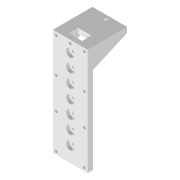
# Autodesk Inventor part: 30_Linear_Captive_Nema8_Base
Saved by Autodesk Inventor 2022 (Build 260153000, 153)
## iProperties
Created: 2022-12-17
Part Number: 30_Linear_Captive_Nema8_Base
Material: Generisch
Document SubType Name: Modeling
Designer: diederichbenedict
Density: 1 g/cm^3
Appearance: Vorgabe
Author: diederichbenedict
Autodesk Inventor part; units mm, degrees
ref_plane "YZ Plane" through (0, 0, 0) normal (1, 0, 0) x (0, 1, 0)
ref_plane "XZ Plane" through (0, 0, 0) normal (0, 1, 0) x (-1, 0, 0)
ref_plane "XY Plane" through (0, 0, 0) normal (0, 0, 1) x (1, 0, 0)
ref_plane "Arbeitsebene1" through (0, 0, 0) normal (0, 0, 1) x (1, 0, 0)
sketch "Skizze1" plane through (0, 0, 0) normal (0, 0, 1) x (1, 0, 0)
  circle A0 centre (0.1, 41.9017) radius 1.75 projected
  circle A1 centre (0.1, 29.4017) radius 1.75 projected
  circle A2 centre (0.1, 16.9017) radius 1.75 projected
  circle A3 centre (0.1, 4.4017) radius 1.75 projected
  line L0 (6.05, 0) -> (-6.05, 0) projected
  line L1 (6.05, 0) -> (6.05, 50) projected
  line L2 (6.05, 50) -> (-6.05, 50) projected
  line L3 (-6.05, 0) -> (-6.05, 50) projected
  line L4 (13.5, 40.6086) -> (13.5, 8.2086) projected
  line L5 (-13.5, 40.6086) -> (-13.5, 8.2086) projected
  line L6 (13.5, -9.8404) -> (-13.3608, -9.8404)
  line L7 (-13.3608, -9.8404) -> (-13.3608, 90.1596)
  line L8 (-13.3608, 90.1596) -> (13.5, 90.1596)
  line L9 (13.5, 90.1596) -> (13.5, -9.8404)
  line L10 (-13.3608, 90.1596) -> (-16.2, 90.1596)
  line L11 (-16.2, 90.1596) -> (-16.2, -9.8404)
  line L12 (-16.2, -9.8404) -> (-13.3608, -9.8404)
  line L13 (-13.3608, -9.8404) -> (-13.3608, 90.1596)
  line L14 (13.5, -9.8404) -> (16.2, -9.8404)
  line L15 (16.2, -9.8404) -> (16.2, 90.1596)
  line L16 (16.2, 90.1596) -> (13.5, 90.1596)
  line L17 (13.5, 90.1596) -> (13.5, -9.8404)
  point P0 (0, 0)
  dimension "d0" = 100
  dimension "d34" = 27
  dimension "d35" = 2.7
  dimension "d36" = 2.7
  constraints: 24 end point, 6 parallel, 3 horizontal, 3 perpendicular, 1 point on line
  measures "d0" distance of L6.end L7.end
  measures "d34" distance from line of L9 L5.start
  measures "d35" distance between parallel lines of L5 L11
  measures "d36" distance between parallel lines of L15 L9
extrude "Extrusion1" add sketch "Skizze1" along normal blind 5 contours A0 | A1 | A2 | A3 | L0 L3 L2 L1 | L9 L16 L15 L14 L4 | L4 L9 L6 L7 L8 | L7 L12 L11 L10
sketch "Skizze2" plane through (0, 0, 0) normal (0, 0, -1) x (-1, 0, 0)
  line L0 (-13.5, 90.1596) -> (16.2, 90.1596)
  line L1 (16.2, 90.1596) -> (-16.2, 90.1596)
  line L2 (-16.2, 90.1596) -> (-16.1921, 85.1596)
  line L3 (-16.1921, 85.1596) -> (16.2, 85.1596)
  line L4 (16.2, 85.1596) -> (16.2, 90.1596)
  line L5 (13.3608, -9.8404) -> (-13.5, -9.8404)
  line L6 (-13.5, -9.8404) -> (-13.5, -4.8404)
  line L7 (-13.5, -4.8404) -> (13.3608, -4.8404)
  line L8 (13.3608, -4.8404) -> (13.3608, -9.8404)
  line L9 (-16.2, 90.1596) -> (16.2, 90.1596) projected
  point P0 (0, 0)
  dimension "d3" = 5
  dimension "d4" = 5
  constraints: 18 end point, 2 coincident, 1 parallel
  measures "d3" distance of L2.end L1.end
  measures "d4" distance of L5.end L6.end
extrude "Extrusion2" add sketch "Skizze2" along normal blind 32 contours L0 L4 L3 L2 L1
sketch "Skizze3" plane through (16.2, -9.8404, 5) normal (1, 0, 0) x (0, 0, -1)
  line L0 (5, 0) -> (5, 95) projected
  line L1 (5, 95) -> (37, 95) projected
  line L2 (37, 100) -> (37, 95) projected
  line L3 (37, 100) -> (0, 100) projected
  line L4 (0, 0) -> (0, 100) projected
  line L5 (37, 100) -> (37, 95) projected
  line L6 (37, 95) -> (5, 80.9723)
  line L7 (5, 95) -> (5, 5) projected
  line L8 (5, 0) -> (0, 0) projected
  point P0 (5, 9.8404)
  constraints: 2 end point, 1 point on line
extrude "Extrusion3" add sketch "Skizze3" against normal blind 5 contours L0 L1 L6
sketch "Skizze4" plane through (-16.2, -9.8404, 5) normal (-1, 0, 0) x (0, 0, 1)
  line L0 (-5, 95) -> (-5, 80.9723) projected
  line L1 (-37, 95) -> (-5, 95) projected
  line L2 (-37, 95) -> (-5, 80.9723) projected
  point P0 (-5, 9.8404)
extrude "Extrusion4" add sketch "Skizze4" against normal blind 5
sketch "Skizze5" plane through (11.2, 85.1596, -32) normal (0, -1, 0) x (1, 0, 0)
  circle A0 centre (-11.2, 4.1) radius 1.75 projected
  point P0 (-11.2, 32)
hole "Bohrung1" at (0, 85.1596, -27.9) direction (0, 1, 0) diameter 3.2 end through all counterbore diameter 6 counterbore depth 3
sketch "Skizze6" plane through (0, 0, 5) normal (0, 0, 1) x (1, 0, 0)
  circle A0 centre (0.1, 16.9017) radius 1.75 projected
  point P0 (0, 0)
hole "Bohrung2" at (0.1, 16.9017, 5) direction (0, 0, -1) diameter 3.2 end through all counterbore diameter 8 counterbore depth 3
pattern_linear "Rechteckige Anordnung1" count 6 spacing 12.5 along (0, 1, 0) count 2 spacing 12.5 along (0, -1, 0) of "Bohrung2"
sketch "Skizze7" plane through (-13.3608, 90.1596, 5) normal (0, 1, 0) x (1, 0, 0)
  arc A0 (19.4108, 9.1706) -> (19.209, 9.3127) centre (19.1621, 9.0317) ccw projected
  arc A1 (18.9122, 9.7059) -> (19.209, 9.3127) centre (19.9951, 10.2147) ccw projected
  arc A2 (18.9122, 9.7059) -> (18.7859, 9.8171) centre (18.694, 9.5854) ccw projected
  line L0 (18.7859, 9.8171) -> (18.2888, 9.8559) projected
  arc A3 (18.0608, 10.0745) -> (18.2888, 9.8559) centre (18.3083, 10.1044) ccw projected
  line L1 (18.0608, 10.0745) -> (18.0608, 10.5256) projected
  arc A4 (18.2884, 10.7739) -> (18.0608, 10.5256) centre (18.3101, 10.5256) ccw projected
  line L2 (18.2884, 10.7739) -> (18.6539, 10.8058) projected
  arc A5 (18.6539, 10.8058) -> (18.9122, 10.9588) centre (18.6817, 11.0536) ccw projected
  arc A6 (19.2562, 11.4767) -> (18.9122, 10.9588) centre (20.0633, 10.5674) ccw projected
  arc A7 (19.2562, 11.4767) -> (19.4108, 11.7) centre (19.1617, 11.7073) ccw projected
  line L3 (19.4108, 11.7) -> (19.4108, 12.3) projected
  line L4 (19.4108, 12.3) -> (18.9108, 12.8) projected
  line L5 (18.9108, 12.8) -> (7.8108, 12.8) projected
  line L6 (7.3108, 12.3) -> (7.8108, 12.8) projected
  line L7 (7.3108, 11.7) -> (7.3108, 12.3) projected
  arc A8 (7.3108, 11.7) -> (7.4655, 11.4767) centre (7.56, 11.7073) ccw projected
  arc A9 (7.8095, 10.9588) -> (7.4655, 11.4767) centre (6.6584, 10.5674) ccw projected
  arc A10 (7.8095, 10.9588) -> (8.0678, 10.8058) centre (8.04, 11.0536) ccw projected
  line L8 (8.4333, 10.7739) -> (8.0678, 10.8058) projected
  arc A11 (8.6608, 10.5256) -> (8.4333, 10.7739) centre (8.4116, 10.5256) ccw projected
  line L9 (8.6608, 10.0745) -> (8.6608, 10.5256) projected
  arc A12 (8.4328, 9.8559) -> (8.6608, 10.0745) centre (8.4134, 10.1044) ccw projected
  line L10 (7.9358, 9.8171) -> (8.4328, 9.8559) projected
  arc A13 (7.9358, 9.8171) -> (7.8095, 9.7059) centre (8.0277, 9.5854) ccw projected
  arc A14 (7.5127, 9.3127) -> (7.8095, 9.7059) centre (6.7266, 10.2147) ccw projected
  arc A15 (7.5127, 9.3127) -> (7.3108, 9.1706) centre (7.5596, 9.0317) ccw projected
  line L11 (7.3108, 5) -> (7.3108, 9.1706) projected
  line L12 (19.4108, 5) -> (7.3108, 5) projected
  line L13 (19.4108, 5) -> (19.4108, 9.1706) projected
  arc A16 (19.9108, 9.2672) -> (19.475, 9.7515) centre (19.1621, 9.0317) ccw
  arc A17 (19.3606, 9.9276) -> (19.475, 9.7515) centre (19.9951, 10.2147) ccw
  arc A18 (19.3606, 9.9276) -> (18.8795, 10.3114) centre (18.694, 9.5854) ccw
  line L14 (18.8795, 10.3114) -> (18.8155, 10.3163)
  arc A19 (18.8155, 10.3163) -> (19.3826, 10.7888) centre (18.6817, 11.0536) ccw
  arc A20 (19.5506, 11.0669) -> (19.3826, 10.7888) centre (20.0633, 10.5674) ccw
  arc A21 (19.5506, 11.0669) -> (19.9108, 11.6946) centre (19.1617, 11.7073) ccw
  line L15 (19.9108, 11.6946) -> (19.9108, 12.5071)
  line L16 (19.9108, 12.5071) -> (19.118, 13.3)
  line L17 (19.118, 13.3) -> (7.6037, 13.3)
  line L18 (7.6037, 13.3) -> (6.8108, 12.5071)
  line L19 (6.8108, 12.5071) -> (6.8108, 11.6946)
  arc A22 (6.8108, 11.6946) -> (7.1711, 11.0669) centre (7.56, 11.7073) ccw
  arc A23 (7.3391, 10.7888) -> (7.1711, 11.0669) centre (6.6584, 10.5674) ccw
  arc A24 (7.3391, 10.7888) -> (7.9062, 10.3163) centre (8.04, 11.0536) ccw
  line L20 (7.9062, 10.3163) -> (7.8422, 10.3114)
  arc A25 (7.8422, 10.3114) -> (7.3611, 9.9276) centre (8.0277, 9.5854) ccw
  arc A26 (7.2467, 9.7515) -> (7.3611, 9.9276) centre (6.7266, 10.2147) ccw
  arc A27 (7.2467, 9.7515) -> (6.8108, 9.2672) centre (7.5596, 9.0317) ccw
  line L21 (6.8108, 9.2672) -> (6.8108, 4.5)
  line L22 (6.8108, 4.5) -> (19.9108, 4.5)
  line L23 (19.9108, 4.5) -> (19.9108, 9.2672)
  point P0 (13.3608, 5)
  dimension "d31" = 0.5
  constraints: 24 point on circle, 20 end point, 12 centre point, 21 other
  measures "d31" distance between parallel lines of L13 L23
extrude "Extrusion5" cut sketch "Skizze7" against normal up to surface (5 mm away) contours L13 L12 L11 A15 A14 A13 L10 A12 L9 A11 L8 A10 A9 A8 L7 L6 L5 L4 L3 A7 A6 A5 L2 A4 L1 A3 L0 A2 A1 A0 | L23 L22 L21 A27 A26 A25 L20 A24 A23 A22 L19 L18 L17 L16 L15 A21 A20 A19 L14 A18 A17 A16
sketch "Skizze10" plane through (0, 0, 5) normal (0, 0, 1) x (1, 0, 0)
  line L0 (16.2, -9.8404) -> (16.2, 90.1596) projected
  line L1 (-16.2, 90.1596) -> (-16.2, -9.8404) projected
  line L2 (16.2, 90.1596) -> (-16.2, 90.1596) projected
  line L3 (-13.2, 54.7596) -> (13.2, 54.7596)
  line L4 (13.2, 54.7596) -> (13.2, 87.1596)
  line L5 (13.2, 87.1596) -> (-13.2, 87.1596)
  line L6 (-13.2, 87.1596) -> (-13.2, 54.7596)
  line L7 (-13.2, 54.7596) -> (13.2, 87.1596) construction
  line L8 (13.2, 54.7596) -> (-13.2, 87.1596) construction
  line L9 (18.5, 39.0086) -> (18.5, 36.2086) projected
  line L10 (17.2, 28.5596) -> (-15.2, 28.5596)
  line L11 (-13.2, -6.8404) -> (13.2, -6.8404)
  line L12 (13.2, -6.8404) -> (13.2, 25.5596)
  line L13 (13.2, 25.5596) -> (-13.2, 25.5596)
  line L14 (-13.2, 25.5596) -> (-13.2, -6.8404)
  line L15 (-13.2, -6.8404) -> (13.2, 25.5596) construction
  line L16 (13.2, -6.8404) -> (-13.2, 25.5596) construction
  line L17 (18.5, 40.6086) -> (18.5, 8.2086) projected
  point P0 (0, 0)
  point P1 (0, 70.9596)
  point P2 (0, 87.1596)
  point P3 (0, 9.3596)
  point P4 (0, 25.5596)
  dimension "d37" = 26.4
  dimension "d38" = 32.4
  dimension "d39" = 3
  dimension "d47" = 26.4
  dimension "d48" = 32.4
  dimension "d49" = 3
  dimension "d50" = 3
  constraints: 26 end point, 6 midpoint, 4 parallel, 2 horizontal, 2 perpendicular
  measures "d37" distance of L5.end L4.end
  measures "d38" distance of L4.end L3.end
  measures "d39" horizontal distance of L0.end L4.end
  measures "d47" distance of L13.end L12.end
  measures "d48" distance of L12.end L11.end
  measures "d49" vertical distance of L10.start L12.end
  measures "d50" horizontal distance of L1.end L11.start
hole "Bohrung3" at (0, 87.1596, 5) at (13.2, 54.7596, 5) at (-13.2, 54.7596, 5) at (-13.2, 87.1596, 5) at (13.2, 87.1596, 5) at (-13.2, -6.8404, 5) at (13.2, -6.8404, 5) at (13.2, 25.5596, 5) at (-13.2, 25.5596, 5) direction (0, 0, -1) diameter 2.8 depth 8 tip angle 118
equation "\"d36\" = d35"
